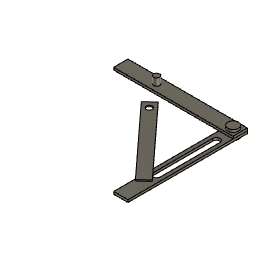
Pin Slot joint (Autodesk Fusion 360 design; units mm, degrees)
Autodesk Fusion 360 part; units mm, degrees
sketch "Sketch1" plane through (0, 0, 0) normal (0, 0, 1) x (1, 0, 0)
  line L0 (0, 0) -> (12, 0)
  line L1 (12, 0) -> (12, 100)
  line L2 (12, 100) -> (0, 100)
  line L3 (0, 100) -> (0, 0)
  line L4 (3, 80) -> (3, 30)
  arc A0 (3, 30) -> (9, 30) centre (6, 30) ccw
  line L5 (9, 30) -> (9, 80)
  arc A1 (9, 80) -> (3, 80) centre (6, 80) ccw
  line L6 (6, 80) -> (6, 30) construction
  line L7 (6, 80) -> (6, 100) construction
  dimension "d1" = 100
  dimension "d2" = 12
  dimension "d3" = 50
  dimension "d4" = 3
  dimension "d5" = 20
  constraint horizontal L0
  constraint vertical L1
  constraint horizontal L2
  constraint vertical L3
  constraint coincident L0.start L3.end
  constraint tangent L4 A0
  constraint tangent A0 L5
  constraint parallel L4 L5
  constraint tangent L5 A1
  constraint tangent L4 A1
  constraint vertical L6
  constraint coincident A1.centre L6.start
  constraint midpoint L2 L7.end
  constraint collinear L6 L7
  measures "d1" distance of L0 L2
  measures "d2" distance of L1 L3
  measures "d3" distance of A1.centre A0.centre
  measures "d4" radius of A0
  measures "d5" vertical distance of A1.centre L7.end
extrude "Extrude1" add sketch "Sketch1" along normal blind 2 makes body 1
sketch "Sketch2" plane through (0, 0, 0) normal (0, 0, 1) x (1, 0, 0)
  line L0 (12, 88) -> (-88, 88)
  line L1 (-88, 88) -> (-88, 100)
  line L2 (-88, 100) -> (12, 100)
  line L3 (12, 100) -> (12, 88)
  line L4 (12, 100) -> (0, 100)
  line L5 (12, 0) -> (12, 100)
  circle A0 centre (6, 94) radius 2.5
  dimension "d8" = 12
  dimension "d9" = 100
  dimension "d10" = 5
  dimension "d11" = 6
  dimension "d12" = 6
  constraint horizontal L0
  constraint vertical L1
  constraint horizontal L2
  constraint vertical L3
  constraint collinear L2 L4
  constraint collinear L3 L5
  measures "d8" distance of L0 L2
  measures "d9" distance of L1.end L2.end
  measures "d10" diameter of A0
  measures "d11" distance of L4 A0.centre
  measures "d12" distance of L5 A0.centre
extrude "Extrude2" add sketch "Sketch2" along normal blind 2 separate body makes body 2
sketch "Sketch3" plane through (0, 0, 2) normal (0, 0, 1) x (-1, 0, 0)
  circle A0 centre (-6, -94) radius 2.5
extrude "Extrude3" cut sketch "Sketch3" against normal through all bodies 1
sketch "Sketch4" plane through (0, 0, 0) normal (0, 0, 1) x (1, 0, 0)
  circle A0 centre (6, 94) radius 2.5
  circle A1 centre (6, 94) radius 4.5
  circle A2 centre (6, 94) radius 2.5
  dimension "d16" = 9
  dimension "d17" = 5
  constraint concentric A0 A1
  constraint concentric A0 A2
  measures "d16" diameter of A1
  measures "d17" diameter of A0
extrude "Extrude4" add sketch "Sketch4" along normal blind 4 and the other way blind 2 separate body contours A0 A2 makes body 3
extrude "Extrude5" add sketch "Sketch4" against normal blind 2 separate body makes body 4
combine "Combine1" operation add target body 3 tool bodies 4
move_body "Move1" bodies 2 to x (1, 0, 0) y (0, 1, 0) z (0, 0, 1) at (0, 0, 2)
sketch "Sketch5" plane through (0, 0, 4) normal (0, 0, 1) x (-1, 0, 0)
  circle A0 centre (-6, -94) radius 4.5
  circle A1 centre (-6, -94) radius 2.5
  dimension "d24" = 9
  constraint concentric A0 A1
  measures "d24" diameter of A0
extrude "Extrude6" add sketch "Sketch5" along normal blind 2 separate body contours A0 | A1 makes body 5
combine "Combine2" operation add target body 5 tool bodies 3
sketch "Sketch6" plane through (0, 0, 4) normal (0, 0, 1) x (-1, 0, 0)
  line L0 (50.5279, -100.7645) -> (43.1532, -107.5183)
  line L1 (43.1532, -107.5183) -> (-10.8773, -48.5208)
  line L2 (-10.8773, -48.5208) -> (-3.5026, -41.767)
  line L3 (-3.5026, -41.767) -> (50.5279, -100.7645)
  circle A0 centre (42.7882, -99.7166) radius 2.5
  circle A1 centre (-3.1377, -49.5687) radius 3
  dimension "d27" = 10
  dimension "d29" = 80
  dimension "d30" = 5
  dimension "d31" = 5
  dimension "d32" = 6
  dimension "d33" = 6
  dimension "d34" = 5
  dimension "d35" = 6
  measures "d27" distance of L1 L3
  measures "d29" distance of L0 L2
  measures "d30" diameter of A0
  measures "d31" distance of L3 A0.centre
  measures "d32" distance of L0 A0.centre
  measures "d33" diameter of A1
  measures "d34" distance of L1 A1.centre
  measures "d35" distance of L2 A1.centre
extrude "Extrude7" add sketch "Sketch6" along normal blind 1 separate body contours L0 L1 L2 L3 | A1 makes body 6
extrude "Extrude8" add sketch "Sketch6" against normal blind 6 separate body contours A1 makes body 7
combine "Combine3" operation add target body 6 tool bodies 7
move_body "Move2" bodies 6 to x (1, 0, 0) y (0, 1, 0) z (0, 0, 1) at (0, -27.0744, 0)
sketch "Sketch7" plane through (0, 0, 4) normal (0, 0, 1) x (-1, 0, 0)
  circle A0 centre (58, -94) radius 2.5
  line L0 (88, -100) -> (88, -88)
  line L1 (88, -88) -> (-12, -88)
  dimension "d40" = 5
  dimension "d41" = 30
  dimension "d42" = 6
  measures "d40" diameter of A0
  measures "d41" distance of A0.centre L0
  measures "d42" distance of A0.centre L1
extrude "Extrude9" add sketch "Sketch7" along normal blind 6 bodies 2
copy_body "Body->Comp1" bodies 1 removing the originals makes body 8 in component "Slot"
copy_body "Body->Comp2" bodies 2 removing the originals makes body 9 in component "Pin arm"
copy_body "Body->Comp3" bodies 6 removing the originals makes body 10 in component "Joint"
copy_body "Body->Comp4" bodies 5 removing the originals makes body 11 in component "Pivot"
component "Slot" placed x (1, 0, 0) y (0, 1, 0) z (0, 0, 1) at (0, 0, 0)
component "Pin arm" placed x (1, 0, 0) y (0, 1, 0) z (0, 0, 1) at (0, 0, 0)
component "Joint" placed x (1, 0, 0) y (0, 1, 0) z (0, 0, 1) at (0, 0, 0)
component "Pivot" placed x (1, 0, 0) y (0, 1, 0) z (0, 0, 1) at (0, 0, 0)
named bodies: "Slot", "Pin arm", "Pivot", "Joint"
